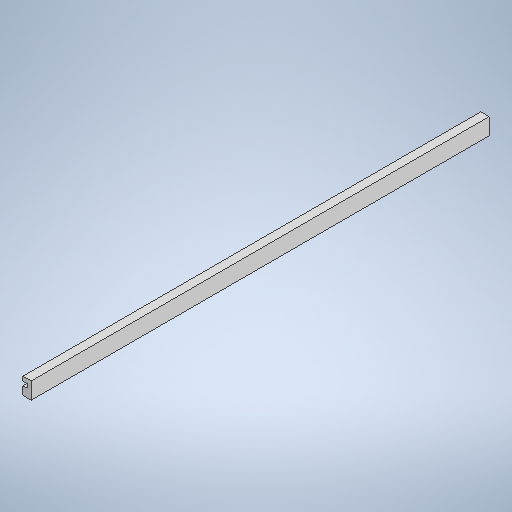
# Autodesk Inventor part: Case Rail
Saved by Autodesk Inventor 2025 (Build 290162000, 162)
## iProperties
Created: 2024-07-16
Part Number: Case Rail
Material: Generic
Document SubType Name: Modeling
Designer: adam
Density: 1 g/cm^3
Appearance: Default
Author: adam
Autodesk Inventor part; units mm, degrees
ref_plane "YZ Plane" through (0, 0, 0) normal (1, 0, 0) x (0, 1, 0)
ref_plane "XZ Plane" through (0, 0, 0) normal (0, 1, 0) x (-1, 0, 0)
ref_plane "XY Plane" through (0, 0, 0) normal (0, 0, 1) x (1, 0, 0)
sketch "Sketch1" plane through (0, 0, 0) normal (0, 0, 1) x (1, 0, 0)
  line L0 (0, 4) -> (2, 4)
  line L1 (2, 4) -> (2, -4)
  line L2 (2, -4) -> (0, -4)
  line L3 (0, -4) -> (0, 4) construction
  line L4 (0, -4) -> (-2, -4)
  line L5 (-2, -4) -> (-2, 0)
  line L6 (-2, 0) -> (0, 0)
  line L7 (0, 0) -> (0, -4)
  line L8 (0, 4) -> (-2, 4)
  line L9 (-2, 4) -> (-2, 1.9)
  line L10 (-2, 1.9) -> (0, 1.9)
  line L11 (0, 1.9) -> (0, 4) construction
  line L12 (0, 1.9) -> (0, 0)
  point P0 (0, 0)
  point P1 (0, 0)
  point P2 (1, 4)
  dimension "d0" = 4
  dimension "d1" = 2
  dimension "d4" = 8
  dimension "d5" = 2
  dimension "d6" = 1.9
  dimension "d7" = 4
  constraints: 26 end point, 6 parallel, 3 horizontal, 3 midpoint, 3 perpendicular, 2 collinear
  measures "d0" distance from line of L2 point (0, 0)
  measures "d1" distance from line of L1 point (0, 0)
  measures "d4" distance between parallel lines of L2 L0
  measures "d5" distance between parallel lines of L3 L5
  measures "d6" distance between parallel lines of L6 L10
  measures "d7" distance of L4.end L5.end
extrude "Extrusion1" add sketch "Sketch1" along normal blind 220
body "Solid1"
